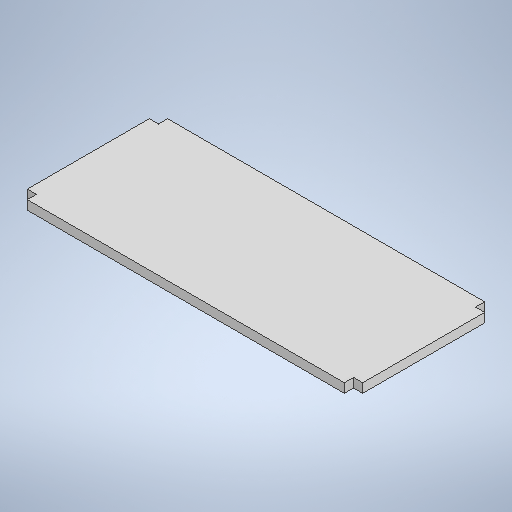
# Autodesk Inventor part: Platform_Arm
Saved by Autodesk Inventor 2025 (Build 290162000, 162)
## iProperties
Created: 2024-06-18
Part Number: Platform_Arm
Material: Generic
Document SubType Name: Modeling
Designer: User
Density: 1 g/cm^3
Appearance: Default
Author: User
Autodesk Inventor part; units mm, degrees
ref_plane "YZ Plane" through (0, 0, 0) normal (1, 0, 0) x (0, 1, 0)
ref_plane "XZ Plane" through (0, 0, 0) normal (0, 1, 0) x (-1, 0, 0)
ref_plane "XY Plane" through (0, 0, 0) normal (0, 0, 1) x (1, 0, 0)
sketch "Sketch1" plane through (0, 0, 0) normal (0, 1, 0) x (-1, 0, 0)
  line L0 (-550, 230) -> (550, 230)
  line L1 (550, 230) -> (550, -230)
  line L2 (550, -230) -> (-550, -230)
  line L3 (-550, -230) -> (-550, 230)
  line L4 (-550, 230) -> (550, -230) construction
  line L5 (550, 230) -> (-550, -230) construction
  point P0 (0, 0)
  dimension "d0" = 1100
  dimension "d1" = 460
  constraints: 12 end point, 2 midpoint, 2 parallel, 1 horizontal, 1 perpendicular
  measures "d0" distance of L1.end L2.end
  measures "d1" distance between parallel lines of L2 L0
extrude "Extrusion1" add sketch "Sketch1" along normal blind 30
sketch "Sketch2" plane through (0, 30, 0) normal (0, 1, 0) x (1, 0, 0)
  line L0 (-550, 230) -> (-550, -230) projected
  line L1 (-550, -230) -> (-520, -230)
  line L2 (-520, -230) -> (-520, -200)
  line L3 (-520, -200) -> (-550, -200)
  line L4 (-550, -200) -> (-550, -230)
  line L5 (-550, 230) -> (-520, 230)
  line L6 (-520, 230) -> (-520, 200)
  line L7 (-520, 200) -> (-550, 200)
  line L8 (-550, 200) -> (-550, 230)
  line L9 (550, -230) -> (550, 230) projected
  line L10 (550, -230) -> (520, -230)
  line L11 (520, -230) -> (520, -200)
  line L12 (520, -200) -> (550, -200)
  line L13 (550, -200) -> (550, -230)
  line L14 (550, 230) -> (520, 230)
  line L15 (520, 230) -> (520, 200)
  line L16 (520, 200) -> (550, 200)
  line L17 (550, 200) -> (550, 230)
  point P0 (0, 0)
  dimension "d6" = 30
  dimension "d7" = 30
  constraints: 32 end point, 8 parallel, 4 equal length, 4 horizontal, 4 perpendicular, 2 point on line
  measures "d6" distance of L1.end L2.end
  measures "d7" distance of L2.end L3.end
extrude "Extrusion2" cut sketch "Sketch2" against normal blind 30
body "Solid1"
